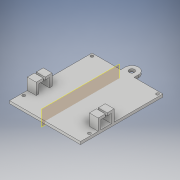
# Autodesk Inventor part: Wheel Base
Saved by Autodesk Inventor 2018 (Build 220112000, 112)
## iProperties
Created: 2018-05-17
Part Number: Wheel Base
Material: Generic
Document SubType Name: Modeling
Designer: alexs
Density: 1 g/cm^3
Appearance: Default
Author: alexs
Autodesk Inventor part; units mm, degrees
ref_plane "YZ Plane" through (0, 0, 0) normal (1, 0, 0) x (0, 1, 0)
ref_plane "XZ Plane" through (0, 0, 0) normal (0, 1, 0) x (-1, 0, 0)
ref_plane "XY Plane" through (0, 0, 0) normal (0, 0, 1) x (1, 0, 0)
sketch "Sketch1" plane through (0, 0, 0) normal (0, 0, 1) x (1, 0, 0)
  line L0 (0, 0) -> (80, 0)
  line L1 (80, 0) -> (80, 93)
  line L2 (80, 93) -> (0, 93)
  line L3 (0, 93) -> (0, 0)
  dimension "d0" = 80
  dimension "d1" = 93
  constraints: 8 end point, 2 parallel, 1 horizontal, 1 perpendicular
  measures "d0" distance of L2.end L1.end
  measures "d1" distance of L1.end L0.end
extrude "Extrusion1" add sketch "Sketch1" along normal blind 3
sketch "Sketch3" plane through (80, 0, 0) normal (1, 0, 0) x (0, 0, -1)
  line L0 (-3, 0) -> (-3, 93) construction
  line L1 (-3, 20) -> (-16, 20)
  line L2 (-16, 38) -> (-3, 38)
  line L3 (-3, 38) -> (-3, 20) construction
  line L4 (-3, 23) -> (-13, 23)
  line L5 (-13, 35) -> (-3, 35)
  line L6 (0, 0) -> (-3, 0) projected
  line L7 (-16, 28) -> (-13, 28)
  line L8 (-13, 30) -> (-16, 30)
  line L9 (-16, 20) -> (-16, 28)
  line L10 (-16, 30) -> (-16, 38)
  line L11 (-13, 23) -> (-13, 28)
  line L12 (-13, 30) -> (-13, 35)
  line L13 (-3, 38) -> (-3, 35)
  line L14 (-3, 20) -> (-3, 23)
  point P0 (-13, 19)
  point P1 (-16, 19)
  dimension "d4" = 3
  dimension "d6" = 20
  dimension "d7" = 12
  dimension "d8" = 10
  dimension "d9" = 3
  dimension "d10" = 5
  dimension "d11" = 5
  dimension "d12" = 3
  constraints: 26 end point, 5 parallel, 5 perpendicular, 3 collinear, 3 horizontal, 3 point on line, 1 horizontal alignment
  measures "d4" distance between parallel lines of L2 L5
  measures "d6" distance between parallel lines of L1 L6
  measures "d7" distance of L4.end L5.start
  measures "d8" distance of L5.start L5.end
  measures "d9" distance of L7.start L7.end
  measures "d10" distance of L4.end L7.end
  measures "d11" distance of L8.start L5.start
  measures "d12" distance between parallel lines of L1 L4
ref_plane "Work Plane1" through (40, 0, 0) normal (1, 0, 0) x (0, 0, -1)
extrude "Extrusion2" add sketch "Sketch3" against normal blind 10
mirror "Mirror1" about plane through (40, 0, 0) normal (1, 0, 0) of "Extrusion2"
sketch "Sketch4" plane through (0, 0, 3) normal (0, 0, 1) x (1, 0, 0)
  circle A0 centre (77, 13) radius 1.6
  line L0 (80, 0) -> (80, 20) projected
  line L1 (0, 0) -> (80, 0) projected
  circle A1 centre (77, 90) radius 1.6
  line L2 (80, 93) -> (0, 93) projected
  dimension "d15" = 3.2
  dimension "d16" = 3
  dimension "d17" = 13
  dimension "d18" = 3
  constraints: 2 centre point, 1 equal radius, 1 vertical alignment
  measures "d15" diameter of A0
  measures "d16" distance from line of L0 A0.centre
  measures "d17" distance from line of L1 A0.centre
  measures "d18" distance from line of L2 A1.centre
extrude "Extrusion3" cut sketch "Sketch4" against normal through all
mirror "Mirror2" about plane through (40, 0, 0) normal (1, 0, 0) of "Extrusion2", "Extrusion3"
sketch "Sketch5" plane through (0, 0, 0) normal (0, 0, -1) x (-1, 0, 0)
  line L0 (-80, 93) -> (0, 93) construction
  line L1 (-47.5, 93) -> (-32.5, 93)
  line L2 (-32.5, 93) -> (-32.5, 98)
  line L3 (-32.5, 98) -> (-47.5, 98) construction
  line L4 (-47.5, 98) -> (-47.5, 93)
  arc A0 (-32.5, 98) -> (-47.5, 98) centre (-40, 98) ccw
  circle A1 centre (-40, 98) radius 3
  point P0 (0, 0)
  point P1 (-40, 93)
  point P2 (-40, 93)
  dimension "d21" = 6
  dimension "d22" = 15
  dimension "d23" = 5
  constraints: 8 end point, 2 centre point, 2 coincident, 2 midpoint, 2 parallel, 2 point on circle, 1 horizontal, 1 perpendicular, 1 point on line, 1 tangent
  measures "d21" diameter of A1
  measures "d22" distance between parallel lines of L2 L4
  measures "d23" distance of L1.end L2.end
extrude "Extrusion4" add sketch "Sketch5" against normal blind 3
equation "\"d11\" = d10"
equation "\"d12\" = d4"
equation "\"d18\" = d16"
equation "\"d5\" = d4"
body "Solid1"
